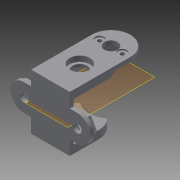
# Autodesk Inventor part: brushless-gearbox
Saved by Autodesk Inventor 2014 SP2 (Build 180247200, 247)
## iProperties
Created: 2018-11-23
Part Number: brushless-gearbox
Material: 一般
Document SubType Name: Modeling
Designer: hide
Density: 1 g/cm^3
Appearance: 既定
Author: hide
Autodesk Inventor part; units mm, degrees
ref_plane "YZ Plane" through (0, 0, 0) normal (1, 0, 0) x (0, 1, 0)
ref_plane "XZ Plane" through (0, 0, 0) normal (0, 1, 0) x (-1, 0, 0)
sketch "スケッチ2" plane through (0, 0, 0) normal (0, 0, 1) x (1, 0, 0)
  circle A0 centre (0, 11) radius 3.8
  circle A1 centre (0, 11) radius 7.25
  line L0 (7.25, 11) -> (7.25, 0)
  line L1 (7.25, 0) -> (-7.25, 0)
  line L2 (-7.25, 0) -> (-7.25, 11)
  circle A2 centre (0, 22.7) radius 2.5
  circle A3 centre (0, 22.7) radius 7.25
  circle A4 centre (-4.25, 22.7) radius 0.75
  circle A5 centre (4.25, 22.7) radius 0.75
  line L3 (7.25, 22.7) -> (7.25, 11)
  line L4 (-7.25, 11) -> (-7.25, 22.7)
  line L5 (-7.25, 11) -> (-3.8, 11)
  line L6 (3.8, 11) -> (7.25, 11)
  line L7 (7.25, 11) -> (3.8, 11)
  line L8 (-3.8, 11) -> (-7.25, 11)
  line L9 (5, 22.7) -> (7.25, 22.7)
  line L10 (-7.25, 22.7) -> (-5, 22.7)
  line L11 (-3.5, 22.7) -> (-2.5, 22.7)
  line L12 (2.5, 22.7) -> (3.5, 22.7)
  point P0 (0, 0)
  dimension "d12" = 14.5
  dimension "d19" = 14.5
  dimension "d11" = 7.6
  dimension "d13" = 14.5
  dimension "d14" = 11
  dimension "d15" = 0
  dimension "d16" = 7.25
  dimension "d17" = 0
  dimension "d18" = 11.7
  dimension "d20" = 5
  dimension "d21" = 8.5
  dimension "d22" = 1.5
  dimension "d23" = 1.5
  dimension "d24" = 4.25
  dimension "d25" = 0
  dimension "d26" = 14.5
  dimension "d27" = 0
  dimension "d28" = 0
  constraints: 26 end point, 12 parallel, 8 point on circle, 6 horizontal, 6 perpendicular, 4 centre point, 2 coincident, 2 horizontal alignment, 4 other
  measures "d11" diameter of A0
  measures "d13" distance between parallel lines of L2 L0
  measures "d14" distance from line of L1 A0.centre
  measures "d15" horizontal distance of point (0, 0) A0.centre
  measures "d16" distance from line of point (0, 0) L2
  measures "d17" distance from line of point (0, 0) L1
  measures "d18" distance of A0.centre A2.centre
  measures "d20" diameter of A2
  measures "d21" distance of A5.centre A4.centre
  measures "d22" diameter of A4
  measures "d23" diameter of A5
  measures "d24" distance of A4.centre A2.centre
  measures "d25" horizontal distance of A0.centre A2.centre
  measures "d26" distance of L4.end L3.start
  measures "d27" vertical distance of A5.centre A4.centre
  measures "d28" vertical distance of A2.centre A4.centre
extrude "押し出し2" add sketch "スケッチ2" along normal blind 3 contours L6 A1 L5 A0 | A0 L5 A1 A3 L6 | L0 L1 L2 A1 | A1 A3 L3 | L4 A3 A1 | A3 A1 | A1 A3 L10 A4 L11 A2 L12 A5 L9 | L9 A5 L12 A2 L11 A4 L10 A3
sketch "スケッチ3" plane through (0, 0, 0) normal (0, 0, -1) x (-1, 0, 0)
  circle A0 centre (0, 11) radius 3.8 projected
  circle A1 centre (0, 11) radius 2.75
  point P0 (0, 0)
  dimension "d31" = 5.5
  constraints: 1 centre point, 1 coincident
  measures "d31" diameter of A1
extrude "押し出し3" add sketch "スケッチ3" against normal blind 1
sketch "スケッチ4" plane through (0, 0, 3) normal (0, 0, 1) x (1, 0, 0)
  circle A0 centre (4.25, 22.7) radius 0.75 projected
  circle A1 centre (-4.25, 22.7) radius 0.75 projected
  circle A2 centre (-4.25, 22.7) radius 1.65
  circle A3 centre (4.25, 22.7) radius 1.65
  point P0 (0, 0)
  dimension "d34" = 3.3
  dimension "d35" = 3.3
  constraints: 2 centre point, 2 coincident
  measures "d34" diameter of A2
  measures "d35" diameter of A3
extrude "押し出し4" cut sketch "スケッチ4" against normal blind 0.5
sketch "スケッチ5" plane through (0, 0, 0) normal (0, 0, -1) x (-1, 0, 0)
  circle A0 centre (-4.25, 22.7) radius 0.75 projected
  circle A1 centre (0, 22.7) radius 2.5 projected
  circle A2 centre (4.25, 22.7) radius 0.75 projected
  arc A3 (7.25, 22.7) -> (-7.25, 22.7) centre (0, 22.7) ccw projected
  line L0 (-7.25, 0) -> (-7.25, 22.7) projected
  line L1 (-7.25, 15.45) -> (7.25, 15.45)
  line L2 (7.25, 15.45) -> (7.25, 29.95)
  line L3 (7.25, 29.95) -> (-7.25, 29.95)
  line L4 (-7.25, 29.95) -> (-7.25, 15.45)
  point P0 (0, 0)
  dimension "d40" = 14.5
  dimension "d41" = 7.25
  constraints: 8 end point, 2 parallel, 1 horizontal, 1 perpendicular, 1 point on line
  measures "d40" distance between parallel lines of L3 L1
  measures "d41" distance from line of A3.centre L3
ref_plane "作業平面1" through (0, 0, -7.4) normal (0, 0, 1) x (1, 0, 0)
mirror "ミラー1" about plane through (0, 0, -7.4) normal (0, 0, 1) of "押し出し2", "押し出し3", "押し出し4"
sketch "スケッチ7" plane through (0, 22.7, -17.8) normal (0, 0, -1) x (-1, 0, 0)
  line L0 (7.25, 0) -> (7.25, -22.7) projected
  arc A0 (7.25, 0) -> (-7.25, 0) centre (0, 0) ccw projected
  line L1 (-7.25, -22.7) -> (-7.25, 0) projected
  circle A1 centre (0, 0) radius 2.5 projected
  circle A2 centre (0, -11.7) radius 3.8 projected
  arc A3 (7.25, -11.7) -> (-7.25, -11.7) centre (0, -11.7) ccw
  point P0 (0, -22.7)
  constraints: 2 point on circle, 2 point on line, 1 centre point, 1 coincident, 1 tangent
extrude "押し出し6" cut sketch "スケッチ7" against normal blind 3 contours L0 A3 L1 A0
sketch "スケッチ8" plane through (0, 0, 0) normal (0, 1, 0) x (-1, 0, 0)
  line L0 (7.25, 0) -> (-7.25, 0) projected
  line L1 (-7.25, 0) -> (-7.25, 3) projected
  line L2 (7.25, 3) -> (-7.25, 3) projected
  line L3 (7.25, 0) -> (7.25, 3) projected
  line L4 (7.25, -14.8) -> (-7.25, -14.8) projected
  line L5 (7.25, -14.8) -> (7.25, -17.8) projected
  line L6 (7.25, -17.8) -> (-7.25, -17.8) projected
  line L7 (-7.25, -14.8) -> (-7.25, -17.8) projected
  line L8 (7.25, 3) -> (-7.25, 3)
  line L9 (-7.25, 3) -> (-7.25, -17.8)
  line L10 (-7.25, -17.8) -> (7.25, -17.8)
  line L11 (7.25, -17.8) -> (7.25, 3)
  line L12 (10, -7.4) -> (-10, -7.4) construction
  line L13 (10, -2.4) -> (-10, -2.4)
  line L14 (-10, -12.4) -> (10, -12.4)
  arc A0 (10, -12.4) -> (10, -2.4) centre (10, -7.4) ccw
  arc A1 (-10, -2.4) -> (-10, -12.4) centre (-10, -7.4) ccw
  circle A2 centre (10, -7.4) radius 1.65
  circle A3 centre (-10, -7.4) radius 1.65
  point P0 (0, 0)
  point P1 (0, -7.4)
  dimension "d45" = 20
  dimension "d46" = 10
  dimension "d47" = 3.3
  dimension "d48" = 3.3
  dimension "d49" = 0
  dimension "d50" = 7.4
  constraints: 16 end point, 4 centre point, 4 parallel, 4 point on circle, 4 tangent, 2 coincident, 1 horizontal, 1 midpoint, 1 perpendicular
  measures "d45" distance of L12.end L12.start
  measures "d46" distance between parallel lines of L14 L13
  measures "d47" diameter of A2
  measures "d48" diameter of A3
  measures "d49" horizontal distance of point (0, -7.4) point (0, 0)
  measures "d50" distance from line of L0 point (0, -7.4)
extrude "押し出し7" add sketch "スケッチ8" along normal blind 1.4 contours L11 L13 L9 L0 | L13 A0 L14 L11 | L11 L14 L9 L13 | L9 L14 A1 L13 | L11 L4 L9 L14
sketch "スケッチ9" plane through (0, 1.4, 0) normal (0, 1, 0) x (1, 0, 0)
  line L0 (7.25, 2.4) -> (10, 2.4) projected
  arc A0 (10, 2.4) -> (10, 12.4) centre (10, 7.4) ccw projected
  arc A1 (-10, 12.4) -> (-10, 2.4) centre (-10, 7.4) ccw projected
  line L1 (-10, 2.4) -> (-7.25, 2.4) projected
  line L2 (-6.6514, 7.4) -> (-8.3257, 4.5)
  line L3 (-8.3257, 4.5) -> (-11.6743, 4.5)
  line L4 (-11.6743, 4.5) -> (-13.3486, 7.4)
  line L5 (-13.3486, 7.4) -> (-11.6743, 10.3)
  line L6 (-11.6743, 10.3) -> (-8.3257, 10.3)
  line L7 (-8.3257, 10.3) -> (-6.6514, 7.4)
  line L8 (-5.4967, 7.4) -> (-7.7483, 3.5)
  line L9 (-7.7483, 3.5) -> (-12.2517, 3.5)
  line L10 (-12.2517, 3.5) -> (-14.5033, 7.4)
  line L11 (-14.5033, 7.4) -> (-12.2517, 11.3)
  line L12 (-12.2517, 11.3) -> (-7.7483, 11.3)
  line L13 (-7.7483, 11.3) -> (-5.4967, 7.4)
  line L14 (13.3486, 7.4) -> (11.6743, 4.5)
  line L15 (11.6743, 4.5) -> (8.3257, 4.5)
  line L16 (8.3257, 4.5) -> (6.6514, 7.4)
  line L17 (6.6514, 7.4) -> (8.3257, 10.3)
  line L18 (8.3257, 10.3) -> (11.6743, 10.3)
  line L19 (11.6743, 10.3) -> (13.3486, 7.4)
  line L20 (14.5033, 7.4) -> (12.2517, 3.5)
  line L21 (12.2517, 3.5) -> (7.7483, 3.5)
  line L22 (7.7483, 3.5) -> (5.4967, 7.4)
  line L23 (5.4967, 7.4) -> (7.7483, 11.3)
  line L24 (7.7483, 11.3) -> (12.2517, 11.3)
  line L25 (12.2517, 11.3) -> (14.5033, 7.4)
  point P0 (0, 0)
  dimension "d53" = 5.8
  dimension "d54" = 5.8
  dimension "d55" = 1
  dimension "d56" = 1
  constraints: 48 end point, 4 coincident, 2 parallel, 52 other
  measures "d53" distance between parallel lines of L3 L6
  measures "d54" distance between parallel lines of L18 L15
  measures "d55" distance between parallel lines of L3 L9
  measures "d56" distance between parallel lines of L15 L21
extrude "押し出し8" add sketch "スケッチ9" along normal blind 1.5
sketch "スケッチ10" plane through (0, 1.4, 0) normal (0, 1, 0) x (1, 0, 0)
  line L0 (7.25, 0) -> (-7.25, 0) projected
  line L1 (-7.25, 14.8) -> (7.25, 14.8) projected
  line L2 (-0.5, 14.8) -> (0.5, 14.8)
  line L3 (0.5, 14.8) -> (0.5, 0)
  line L4 (0.5, 0) -> (-0.5, 0)
  line L5 (-0.5, 0) -> (-0.5, 14.8)
  point P0 (0, 0)
  dimension "d59" = 1
  dimension "d60" = 0.5
  constraints: 8 end point, 2 parallel, 2 point on line, 1 horizontal, 1 perpendicular
  measures "d59" distance between parallel lines of L3 L5
  measures "d60" distance from line of point (0, 0) L5
extrude "押し出し9" add sketch "スケッチ10" along normal blind 6
extrude "押し出し10" cut sketch "スケッチ5" against normal blind 1.4
chamfer "面取り1" distance 1.4 angle 45 1 edges at (0, 15.45, 1.4)
sketch "スケッチ12" plane through (7.25, 0, -17.8) normal (0, 0, -1) x (-1, 0, 0)
  circle A0 centre (7.25, 22.7) radius 2.5 projected
  circle A1 centre (7.25, 22.7) radius 6.25
  point P0 (7.25, 0)
  dimension "d69" = 12.5
  constraints: 1 centre point, 1 coincident
  measures "d69" diameter of A1
extrude "押し出し11" cut sketch "スケッチ12" against normal blind 3
chamfer "面取り2" distance 2 angle 45 1 edges at (0, 16.45, -14.8)
sketch "スケッチ14" plane through (0, 0, 1.4) normal (0, 0, -1) x (-1, 0, 0)
  circle A0 centre (-4.25, 22.7) radius 0.75 projected
  circle A1 centre (4.25, 22.7) radius 0.75 projected
  circle A2 centre (0, 22.7) radius 2.5 projected
  arc A3 (7.25, 22.7) -> (-7.25, 22.7) centre (0, 22.7) ccw projected
  circle A4 centre (0, 22.7) radius 6.75
  point P0 (0, 0)
  dimension "d75" = 13.5
  constraints: 1 centre point, 1 coincident
  measures "d75" diameter of A4
extrude "押し出し12" cut sketch "スケッチ14" along normal blind 10
fillet "フィレット1" radius 2 1 edges at (0, 15.95, 0.5001)
sketch "スケッチ15" plane through (0.5, 1.4, 0) normal (1, 0, 0) x (0, 0, -1)
  circle A0 centre (2.4, 3) radius 1.5
  circle A1 centre (7.4, 3) radius 1.5
  circle A2 centre (12.4, 3) radius 1.5
  line L0 (7.4, 0) -> (7.4, 1.5) projected
  point P0 (0, -1.4)
  dimension "d79" = 3
  dimension "d80" = 3
  dimension "d81" = 3
  dimension "d82" = 5
  dimension "d83" = 5
  dimension "d84" = 0
  constraints: 3 centre point
  measures "d79" diameter of A1
  measures "d80" diameter of A0
  measures "d81" diameter of A2
  measures "d82" distance of A1.centre A0.centre
  measures "d83" distance of A1.centre A2.centre
  measures "d84" distance from line of L0 A1.centre
extrude "押し出し13" cut sketch "スケッチ15" against normal blind 1
equation "\"d12\" = d19"
equation "\"d13\" = d12"
equation "\"d16\" = 0.5 * d13"
equation "\"d23\" = d22"
equation "\"d24\" = 0.5 * d21"
equation "\"d26\" = d19"
equation "\"d35\" = d34"
equation "\"d41\" = 0.5 * d40"
equation "\"d48\" = d47"
equation "\"d54\" = d53"
equation "\"d56\" = d55"
equation "\"d60\" = 0.5 * d59"
equation "\"d80\" = d79"
equation "\"d81\" = d79"
equation "\"d83\" = d82"
